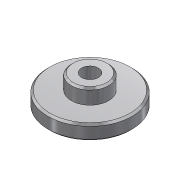
# Autodesk Inventor part: BC-10011
Saved by Autodesk Inventor 2016 (Build 200138000, 138)
## iProperties
Created: 2015-11-26
Part Number: BC-10011
Project: DIPOLO BC-3T- SIRIUS
Cost Center: 1504002005
Material: Aço Inox AISI 304
Document SubType Name: Modeling
Designer: reinaldo.basilio
Density: 8 g/cm^3
Appearance: Chrome - Satin
Description: Calibrador angular.
Mass: 14.0515 g
Surface Area: 12.3349 cm^2
Volume: 1.75643 cm^3
RuleStatus: InUse
AfterMaterialChange0: file://_iMaterial
AfterAnyiPropertyChange0: file://_iMaterial
AfterDocNew0: file://_Naming_par
AfterDocNew1: file://_NameStart
AfterDocNew2: file://_NameStart1
AfterDocNew3: file://_Materiais
DocNumber: XXXXX-XXX-XXXX-00-001.ipt
Folder: .
Title: DIPOLO BC-3T- SIRIUS
Author: reinaldo.basilio
Subject: BC-10011
Autodesk Inventor part; units mm, degrees
ref_plane "YZ Plane" through (0, 0, 0) normal (1, 0, 0) x (0, 1, 0)
ref_plane "XZ Plane" through (0, 0, 0) normal (0, 1, 0) x (-1, 0, 0)
ref_plane "XY Plane" through (0, 0, 0) normal (0, 0, 1) x (1, 0, 0)
sketch "Sketch5" plane through (0, 0, 0) normal (0, 0, 1) x (1, 0, 0)
  circle A0 centre (0, 0) radius 11.251
  dimension "d8" = 22.502
  constraints: 1 centre point, 1 coincident
  measures "d8" diameter of A0
extrude "Extrusion5" add sketch "Sketch5" along normal blind 4
sketch "Sketch6" plane through (0, 0, 4) normal (0, 0, 1) x (1, 0, 0)
  circle A0 centre (0, 0) radius 11.251 projected
  circle A1 centre (0, 0) radius 5
  dimension "d15" = 10
  constraints: 1 centre point, 1 coincident
  measures "d15" diameter of A1
extrude "Extrusion6" add sketch "Sketch6" along normal blind 4 contours A1
hole "Hole1" at (0, 0, 0) direction (0, 0, 1) diameter 4.5 end through all
chamfer "Chamfer2" distance 0.5 angle 45 3 edges at (-11.251, 0, 0) (-11.251, 0, 4) (-5, 0, 8)
body "Solid5"
